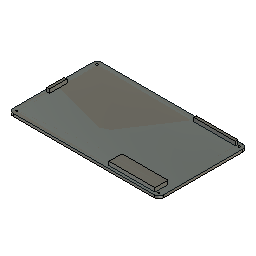
Thermal_printer_down v2 (Autodesk Fusion 360 design; units mm, degrees)
Autodesk Fusion 360 part; units mm, degrees
sketch "Sketch1" plane through (0, 0, 0) normal (0, 0, 1) x (1, 0, 0)
  line L0 (5, 0) -> (165, 0)
  line L1 (170, 5) -> (170, 95)
  line L2 (165, 100) -> (5, 100)
  line L3 (0, 95) -> (0, 5)
  arc A0 (0, 5) -> (5, 0) centre (5, 5) ccw
  arc A1 (5, 100) -> (0, 95) centre (5, 95) ccw
  arc A2 (170, 95) -> (165, 100) centre (165, 95) ccw
  arc A3 (165, 0) -> (170, 5) centre (165, 5) ccw
  point P0 (170, 0)
  point P1 (0, 100)
  dimension "d1" = 170
  dimension "d2" = 100
  dimension "d3" = 5
  dimension "d4" = 5
  dimension "d5" = 5
  dimension "d6" = 5
  constraint horizontal L0
  constraint vertical L1
  constraint horizontal L2
  constraint vertical L3
  constraint coincident origin L3
  constraint coincident origin L0
  constraint tangent L3 A0
  constraint tangent L0 A0
  constraint coincident P1 L3
  constraint coincident P1 L2
  constraint tangent L3 A1
  constraint tangent L2 A1
  constraint tangent L2 A2
  constraint tangent L1 A2
  constraint coincident P0 L0
  constraint coincident P0 L1
  constraint tangent L0 A3
  constraint tangent L1 A3
  measures "d1" distance of origin P0
  measures "d2" distance of origin P1
  measures "d3" radius of A0
  measures "d4" radius of A1
  measures "d5" radius of A2
  measures "d6" radius of A3
extrude "Extrude1" add sketch "Sketch1" along normal blind 3
sketch "Sketch2" plane through (0, 0, 3) normal (0, 0, 1) x (-1, 0, 0)
  arc A0 (-165, 0) -> (-170, -5) centre (-165, -5) ccw
  line L0 (-170, -5) -> (-170, -95)
  arc A1 (-170, -95) -> (-165, -100) centre (-165, -95) ccw
  line L1 (-165, -100) -> (-5, -100)
  arc A2 (-5, -100) -> (0, -95) centre (-5, -95) ccw
  line L2 (0, -95) -> (0, -5)
  arc A3 (0, -5) -> (-5, 0) centre (-5, -5) ccw
  line L3 (-5, 0) -> (-165, 0)
  line L4 (-3, -95) -> (-3, -5)
  arc A4 (-3, -5) -> (-5, -3) centre (-5, -5) ccw
  line L5 (-5, -3) -> (-165, -3)
  arc A5 (-165, -3) -> (-167, -5) centre (-165, -5) ccw
  line L6 (-167, -5) -> (-167, -95)
  arc A6 (-167, -95) -> (-165, -97) centre (-165, -95) ccw
  arc A7 (-5, -97) -> (-3, -95) centre (-5, -95) ccw
  line L7 (-7.5, -92.5) -> (-7.5, -7.5)
  line L8 (-7.5, -7.5) -> (-110.5, -7.5)
  line L9 (-162.5, -7.5) -> (-162.5, -92.5)
  line L10 (-162.5, -92.5) -> (-7.5, -92.5)
  line L11 (-162.5, -92.5) -> (-162.5, -97)
  line L12 (-162.5, -92.5) -> (-98.5, -92.5)
  line L13 (-98.5, -92.5) -> (-98.5, -97)
  line L14 (-115.5, -97) -> (-162.5, -97)
  line L15 (-162.5, -97) -> (-162.5, -92.5)
  line L16 (-162.5, -7.5) -> (-162.5, -3)
  line L17 (-162.5, -3) -> (-110.5, -3)
  line L18 (-110.5, -3) -> (-110.5, -14.36)
  line L19 (-110.5, -14.36) -> (-162.5, -14.36)
  line L20 (-162.5, -14.36) -> (-162.5, -3)
  line L21 (-115.5, -97) -> (-162.5, -97)
  line L22 (-162.5, -97) -> (-162.5, -94)
  line L23 (-162.5, -94) -> (-115.5, -94)
  line L24 (-98.5, -94) -> (-98.5, -97)
  line L25 (-162.5, -94) -> (-115.5, -94)
  line L26 (-115.5, -94) -> (-115.5, -97)
  line L27 (-115.5, -97) -> (-162.5, -97)
  line L28 (-162.5, -97) -> (-162.5, -94)
  line L29 (-165, -97) -> (-115.5, -97)
  line L30 (-98.5, -97) -> (-5, -97)
  dimension "d11" = 64
  dimension "d12" = 52
  dimension "d13" = 11.36
  dimension "d14" = 3
  dimension "d15" = 47
  constraint coincident L11.end L29
  constraint perpendicular L11 L29
  constraint horizontal L12
  constraint vertical L13
  constraint horizontal L14
  constraint vertical L15
  constraint coincident L5 L16.end
  constraint perpendicular L5 L16
  constraint horizontal L17
  constraint vertical L18
  constraint horizontal L19
  constraint vertical L20
  constraint horizontal L21
  constraint vertical L22
  constraint horizontal L23
  constraint vertical L24
  constraint coincident L18 L8.end
  constraint horizontal L25
  constraint vertical L26
  constraint horizontal L27
  constraint vertical L28
  constraint concentric A3 A4
  constraint concentric A0 A5
  constraint concentric A1 A6
  constraint concentric A2 A7
  constraint tangent L4 A7
  constraint tangent A5 L6
  constraint tangent L4 A4
  constraint tangent A4 L5
  constraint tangent L5 A5
  constraint tangent L6 A6
  constraint tangent A6 L29
  constraint tangent A7 L29
  constraint collinear L29 L30
  measures "d11" distance of L9.end L12.end
  measures "d12" distance of L16.end L17.end
  measures "d13" distance of L16.end L19.end
  measures "d14" distance of L13.end L24.start
  measures "d15" distance of L22.end L23.end
extrude "Extrude2" add sketch "Sketch2" along normal blind 4.3 contours L5 L9 L16 L17 L18 L19 L20 | L11 L14 L15 L21 L22 L23 L25 L26 L27 L28 L29
sketch "Sketch3" plane through (0, 0, 3) normal (0, 0, 1) x (-1, 0, 0)
  line L0 (-162.5, -97) -> (-162.5, -94)
  line L1 (-162.5, -94) -> (-115.5, -94)
  line L2 (-115.5, -94) -> (-115.5, -97)
  line L3 (-115.5, -97) -> (-162.5, -97)
  line L4 (-162.5, -14.36) -> (-162.5, -3)
  line L5 (-162.5, -3) -> (-110.5, -3)
  line L6 (-110.5, -3) -> (-110.5, -14.36)
  line L7 (-110.5, -14.36) -> (-162.5, -14.36)
  arc A0 (-165, 0) -> (-170, -5) centre (-165, -5) ccw
  line L8 (-170, -5) -> (-170, -95)
  arc A1 (-170, -95) -> (-165, -100) centre (-165, -95) ccw
  line L9 (-165, -100) -> (-5, -100)
  arc A2 (-5, -100) -> (0, -95) centre (-5, -95) ccw
  line L10 (0, -95) -> (0, -5)
  arc A3 (0, -5) -> (-5, 0) centre (-5, -5) ccw
  line L11 (-5, 0) -> (-165, 0)
sketch "Sketch4" plane through (0, 0, 3) normal (0, 0, 1) x (1, 0, 0)
extrude "Extrude3" add 1 faces at (127.8333, 14.36, 4.4333) along direction (0, 1, 0) blind 3.34
sketch "Sketch5" plane through (0, 0, 3) normal (0, 0, 1) x (-1, 0, 0)
sketch "Sketch6" plane through (0, 0, 3) normal (0, 0, 1) x (-1, 0, 0)
  circle A0 centre (-4.5302, -4.5302) radius 1
  circle A1 centre (-4.5302, -95.4698) radius 1
  circle A2 centre (-165.4698, -95.4698) radius 1
  circle A3 centre (-165.4698, -4.5302) radius 1
  dimension "d26" = 2
  dimension "d30" = 2
  dimension "d34" = 2
  dimension "d38" = 2
  measures "d26" diameter of A0
  measures "d30" diameter of A1
  measures "d34" diameter of A2
  measures "d38" diameter of A3
extrude "Extrude4" cut sketch "Sketch6" against normal blind 3
sketch "Sketch7" plane through (0, 0, 0) normal (0, 0, -1) x (1, 0, 0)
  circle A0 centre (4.5302, -95.4698) radius 1
  circle A1 centre (165.4698, -95.4698) radius 1
  circle A2 centre (4.5302, -4.5302) radius 1
  circle A3 centre (165.4698, -4.5302) radius 1
  arc A4 (170, -5) -> (165, 0) centre (165, -5) ccw
  line L0 (165, 0) -> (5, 0)
  arc A5 (5, 0) -> (0, -5) centre (5, -5) ccw
  line L1 (0, -5) -> (0, -95)
  arc A6 (0, -95) -> (5, -100) centre (5, -95) ccw
  line L2 (5, -100) -> (165, -100)
  arc A7 (165, -100) -> (170, -95) centre (165, -95) ccw
  line L3 (170, -95) -> (170, -5)
  circle A8 centre (4.5302, -4.5302) radius 2.5
  circle A9 centre (4.5302, -95.4698) radius 2.5
  circle A10 centre (165.4698, -95.4698) radius 2.5
  circle A11 centre (165.4698, -4.5302) radius 2.5
  dimension "d41" = 1.5
  dimension "d42" = 1.5
  dimension "d43" = 1.5
  dimension "d44" = 1.5
extrude "Extrude5" cut sketch "Sketch7" against normal blind 1 contours A8 | A9 | A10 | A11
sketch "Sketch8" plane through (0, 0, 3) normal (0, 0, 1) x (1, 0, 0)
sketch "Sketch9" plane through (0, 0, 3) normal (0, 0, 1) x (-1, 0, 0)
  line L0 (-3, -40) -> (-6, -40)
  line L1 (-6, -40) -> (-6, -60)
  line L2 (-6, -60) -> (-3, -60)
  line L3 (-3, -60) -> (-3, -40)
  point P0 (-4.5, -50)
  dimension "d51" = 3
  dimension "d52" = 20
  constraint horizontal L0
  constraint perpendicular L0 L1
  constraint parallel L0 L2
  constraint parallel L1 L3
  measures "d51" distance of L1.end L2.end
  measures "d52" distance of L0.end L1.end
extrude "Extrude6" add sketch "Sketch9" along normal blind 4.3
